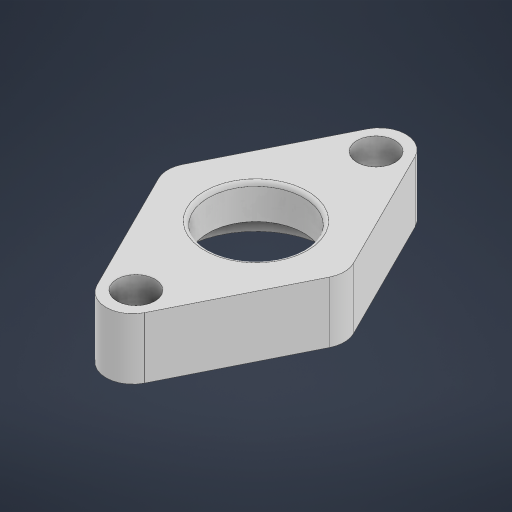
# Autodesk Inventor part: no-filter-inlet
Saved by Autodesk Inventor 2024.2 (Build 282272000, 272)
## iProperties
Created: 2025-06-20
Part Number: no-filter-inlet
Material: Generic
Document SubType Name: Modeling
Designer: Moe
Density: 1 g/cm^3
Appearance: Default
Author: Moe
Autodesk Inventor part; units mm, degrees
ref_plane "YZ Plane" through (0, 0, 0) normal (1, 0, 0) x (0, 1, 0)
ref_plane "XZ Plane" through (0, 0, 0) normal (0, 1, 0) x (-1, 0, 0)
ref_plane "XY Plane" through (0, 0, 0) normal (0, 0, 1) x (1, 0, 0)
sketch "Sketch1" plane through (0, 0, 0) normal (0, 1, 0) x (-1, 0, 0)
  circle A0 centre (0, 0) radius 6.25
  circle A1 centre (0, -15.75) radius 2.5
  circle A2 centre (0, 15.75) radius 2.5
  line L0 (0, 0) -> (0, -24)
  line L1 (0, 0) -> (0, 24)
  line L2 (0, 0) -> (12, 0)
  line L3 (0, 0) -> (-12, 0)
  line L4 (0, 24) -> (12, 0)
  line L5 (12, 0) -> (0, -24)
  line L6 (0, -24) -> (-12, 0)
  line L7 (-12, 0) -> (0, 24)
  dimension "d0" = 12.5
  dimension "d1" = 5
  dimension "d2" = 5
  dimension "d3" = 15.75
  dimension "d4" = 15.75
  dimension "d5" = 24
  dimension "d6" = 24
  dimension "d7" = 12
  dimension "d8" = 12
  constraints: 16 end point, 3 centre point, 2 horizontal, 2 vertical, 1 coincident
  measures "d0" diameter of A0
  measures "d1" diameter of A1
  measures "d2" diameter of A2
  measures "d3" distance of point (0, 0) A2.centre
  measures "d4" distance of A1.centre point (0, 0)
  measures "d5" distance of L0.start L0.end
  measures "d6" distance of L0.start L1.end
  measures "d7" distance of L0.start L2.end
  measures "d8" distance of L0.start L3.end
extrude "Extrusion1" add sketch "Sketch1" along normal blind 8 contours L2 L5 L0 A1 A0 | A0 L1 A2 L4 L2 | A0 L3 L7 L1 A2 | L0 A1 L6 L3 A0
fillet "Fillet1" radius 3.5 4 edges at (0, 4, 24) (0, 4, -24) (12, 4, 0) (-12, 4, 0)
sketch "Sketch2" plane through (0, 0, 0) normal (0, -1, 0) x (1, 0, 0)
  circle A0 centre (0, 0) radius 6.25 projected
  circle A1 centre (0, 0) radius 9.625
  dimension "d12" = 19.25
  constraints: 1 centre point, 1 coincident
  measures "d12" diameter of A1
extrude "Extrusion2" cut sketch "Sketch2" against normal blind 3.5
fillet "Fillet2" radius 0.5 1 edges at (6.25, 8, 0)
body "Solid1"
